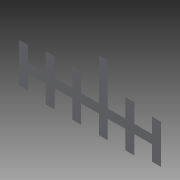
# Autodesk Inventor part: Trigger_Copper
Saved by Autodesk Inventor 2014 SP1 (Build 180222100, 222)
## iProperties
Created: 2014-01-12
Part Number: Trigger_Copper
Material: Copper
Document SubType Name: Modeling
Designer: tuleu
Density: 8.94 g/cm^3
Appearance: Copper - Satin
Author: tuleu
Autodesk Inventor part; units mm, degrees
ref_plane "YZ Plane" through (0, 0, 0) normal (1, 0, 0) x (0, 1, 0)
ref_plane "XZ Plane" through (0, 0, 0) normal (0, 1, 0) x (-1, 0, 0)
ref_plane "XY Plane" through (0, 0, 0) normal (0, 0, 1) x (1, 0, 0)
sketch "Sketch1" plane through (0, 0, 0) normal (0, 1, 0) x (-1, 0, 0)
  line L0 (87.5, 6.25) -> (87.5, 27.5)
  line L1 (87.5, 27.5) -> (100, 27.5)
  line L2 (100, 27.5) -> (100, -27.5)
  line L3 (100, -27.5) -> (87.5, -27.5)
  line L4 (87.5, -27.5) -> (87.5, -6.25)
  line L5 (0, 31.6943) -> (0, -31.6996)
  line L6 (0, 0) -> (100, 0)
  line L7 (-87.5, 6.25) -> (-87.5, 27.5)
  line L8 (-87.5, 27.5) -> (-100, 27.5)
  line L9 (-100, 27.5) -> (-100, -27.5)
  line L10 (-100, -27.5) -> (-87.5, -27.5)
  line L11 (-87.5, -27.5) -> (-87.5, -6.25)
  line L12 (62.5, -32.5) -> (50, -32.5)
  line L13 (50, 32.5) -> (62.5, 32.5)
  line L14 (62.5, 32.5) -> (62.5, 6.25)
  line L15 (62.5, -6.25) -> (62.5, -32.5)
  line L16 (87.5, -6.25) -> (62.5, -6.25)
  line L17 (50, -32.5) -> (50, -6.25)
  line L18 (50, 6.25) -> (50, 32.5)
  line L19 (62.5, 6.25) -> (87.5, 6.25)
  line L20 (25, -32.5) -> (12.5, -32.5)
  line L21 (12.5, 32.5) -> (25, 32.5)
  line L22 (25, 32.5) -> (25, 6.25)
  line L23 (25, -6.25) -> (25, -32.5)
  line L24 (12.5, -32.5) -> (12.5, -6.25)
  line L25 (12.5, 6.25) -> (12.5, 32.5)
  line L26 (-12.5, -32.5) -> (-25, -32.5)
  line L27 (-25, 65) -> (-12.5, 65)
  line L28 (-50, -32.5) -> (-62.5, -32.5)
  line L29 (-50, -6.25) -> (-50, -32.5)
  line L30 (-62.5, -32.5) -> (-62.5, -6.25)
  line L31 (-50, 32.5) -> (-50, 6.25)
  line L32 (-62.5, 6.25) -> (-62.5, 32.5)
  line L33 (-62.5, 32.5) -> (-50, 32.5)
  line L34 (50, -6.25) -> (25, -6.25)
  line L35 (12.5, -6.25) -> (0, -6.25)
  line L36 (0, 6.25) -> (12.5, 6.25)
  line L37 (25, 6.25) -> (50, 6.25)
  line L38 (0, 6.25) -> (-12.5, 6.25)
  line L39 (-12.5, -6.25) -> (0, -6.25)
  line L40 (-87.5, -6.25) -> (-62.5, -6.25)
  line L41 (-50, -6.25) -> (-25, -6.25)
  line L42 (-25, 6.25) -> (-50, 6.25)
  line L43 (-62.5, 6.25) -> (-87.5, 6.25)
  line L44 (-12.5, 65) -> (-12.5, 6.25)
  line L45 (-12.5, -6.25) -> (-12.5, -32.5)
  line L46 (-25, -32.5) -> (-25, -6.25)
  line L47 (-25, 6.25) -> (-25, 65)
  dimension "d1" = 55
  dimension "d2" = 12.5
  dimension "d4" = 100
  dimension "d5" = 65
  dimension "d7" = 25
  dimension "d8" = 12.5
  dimension "d11" = 37.5
  dimension "d17" = 97.5
  dimension "d18" = 12.5
  dimension "d21" = 75
  dimension "d26" = 25
  constraints: 96 end point, 27 parallel, 14 collinear, 11 perpendicular, 7 horizontal, 6 symmetric about line, 3 point on line, 1 midpoint, 31 other
  measures "d1" distance of L1.end L2.end
  measures "d2" distance of L2.end L3.end
  measures "d4" distance from line of L6.start L2
  measures "d5" distance of L13.end L12.start
  measures "d7" distance between parallel lines of L4 L15
  measures "d8" distance between parallel lines of L19 L16
  measures "d11" distance of L12.start L20.start
  measures "d17" distance between parallel lines of L27 L26
  measures "d18" distance of L26.start L26.end
  measures "d21" distance of L23.start L29.start
  measures "d26" distance between parallel lines of L45 L24
extrude "Extrusion1" add sketch "Sketch1" along normal blind 0.01
body "Solid1"
